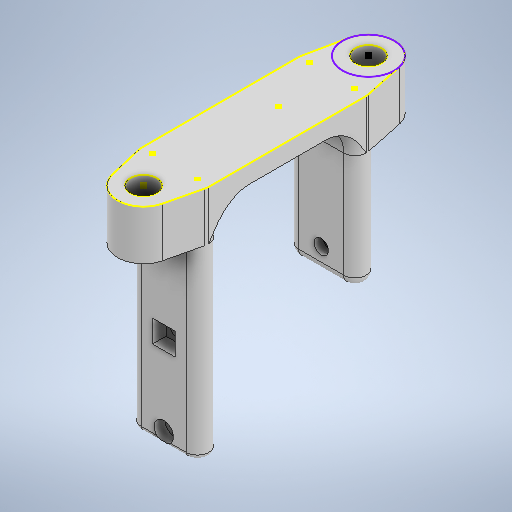
# Autodesk Inventor part: Latest_Odom
Saved by Autodesk Inventor 2025.1 (Build 291241020, 241B)
## iProperties
Created: 2024-11-18
Part Number: Latest_Odom
Material: Generic
Document SubType Name: Modeling
Designer: colli
Density: 1 g/cm^3
Appearance: Default
Author: colli
Autodesk Inventor part; units mm, degrees
ref_plane "YZ Plane" through (0, 0, 0) normal (1, 0, 0) x (0, 1, 0)
ref_plane "XZ Plane" through (0, 0, 0) normal (0, 1, 0) x (-1, 0, 0)
ref_plane "XY Plane" through (0, 0, 0) normal (0, 0, 1) x (1, 0, 0)
sketch "Sketch1" plane through (0, 0, 0) normal (0, 1, 0) x (-1, 0, 0)
  line L0 (1.833087, 41.275) -> (-1.833087, 41.275)
  line L1 (-1.833087, 41.275) -> (-3.666174, 38.1)
  line L2 (-3.666174, 38.1) -> (-1.833087, 34.925)
  line L3 (-1.833087, 34.925) -> (1.833087, 34.925)
  line L4 (1.833087, 34.925) -> (3.666174, 38.1)
  line L5 (3.666174, 38.1) -> (1.833087, 41.275)
  circle A0 centre (0, 38.1) radius 2.0955
  circle A1 centre (0, 38.1) radius 3.0353
  arc A2 (6.01682, 40.129871) -> (-6.01682, 40.129871) centre (0, 38.1) ccw
  line L6 (9.525, 29.21) -> (9.525, -15.24)
  line L7 (-9.525, 29.21) -> (-9.525, 19.812)
  circle A3 centre (0, 38.1) radius 3.81
  line L8 (-9.525, 19.812) -> (-9.525, 6.35)
  line L9 (9.525, 19.812) -> (9.525, 6.35)
  line L10 (0, 19.812) -> (0, -7.112) construction
  line L11 (0, 38.1) -> (0, 31.75)
  line L12 (9.525, -15.24) -> (9.525, 6.35)
  line L13 (-9.525, -15.24) -> (-9.525, 6.35)
  line L14 (1.833087, -28.575) -> (-1.833087, -28.575)
  line L15 (-1.833087, -28.575) -> (-3.666174, -25.4)
  line L16 (-3.666174, -25.4) -> (-1.833087, -22.225)
  line L17 (-1.833087, -22.225) -> (1.833087, -22.225)
  line L18 (1.833087, -22.225) -> (3.666174, -25.4)
  line L19 (3.666174, -25.4) -> (1.833087, -28.575)
  circle A4 centre (0, -25.4) radius 2.0955
  circle A5 centre (0, -25.4) radius 3.0353
  arc A6 (-6.01682, -27.429871) -> (6.01682, -27.429871) centre (0, -25.4) ccw
  line L20 (6.35, -12.065) -> (-6.35, -12.065)
  arc A7 (-6.35, -12.065) -> (-6.35, -18.415) centre (-6.35, -15.24) ccw
  arc A8 (6.35, -18.415) -> (6.35, -12.065) centre (6.35, -15.24) ccw
  line L21 (9.525, -15.24) -> (9.525, -7.112)
  line L22 (-9.525, -15.24) -> (-9.525, -7.112)
  circle A9 centre (0, -25.4) radius 3.81
  line L23 (0, -25.4) -> (0, -19.05)
  line L24 (6.35, -18.415) -> (-6.35, -18.415)
  line L25 (-6.01682, -27.429871) -> (-9.391765, -16.150106)
  line L26 (6.01682, -27.429871) -> (9.391765, -16.150106)
  line L27 (0, 31.115) -> (0, 32.385)
  line L28 (0, 32.385) -> (-6.35, 32.385)
  line L29 (0, 32.385) -> (6.35, 32.385)
  arc A10 (-6.35, 32.385) -> (-6.35, 26.035) centre (-6.35, 29.21) ccw
  line L30 (-6.35, 26.035) -> (6.35, 26.035)
  arc A11 (6.35, 26.035) -> (6.35, 32.385) centre (6.35, 29.21) ccw
  line L31 (-6.01682, 40.129871) -> (-9.35841, 30.224936)
  line L32 (6.01682, 40.129871) -> (9.35841, 30.224936)
  point P0 (0, 0)
  point P1 (-9.525, -16.51)
  point P2 (9.525, -16.51)
  dimension "d35" = 7.62
  dimension "d91" = 6.35
  dimension "d120" = 1.27
  constraints: 68 end point, 12 point on circle, 10 centre point, 5 tangent, 4 coincident, 2 horizontal, 2 point on line, 1 vertical, 12 other
  measures "d35" diameter of A3
  measures "d91" distance of L11.start L11.end
  measures "d120" distance of L27.start L27.end
extrude "Extrusion18" add sketch "Sketch1" along normal blind 5.08 contours A8 L24 A7 L20 | L26 A6 L25 A7 L24 A8
extrude "Extrusion19" add sketch "Sketch1" against normal blind 41.275 contours A8 L24 A7 L20
sketch "Sketch14" plane through (0, -41.275, 0) normal (0, -1, 0) x (1, 0, 0)
  arc A0 (-6.35, 31.115) -> (-6.35, 24.765) centre (-6.35, 27.94) ccw projected
  line L0 (-6.35, 24.765) -> (6.35, 24.765) projected
  arc A1 (6.35, 24.765) -> (6.35, 31.115) centre (6.35, 27.94) ccw projected
  line L1 (6.35, 31.115) -> (-6.35, 31.115) projected
  point P0 (0, 0)
extrude "Extrusion23" add sketch "Sketch14" along normal blind 20.472933
extrude "Extrusion26" add sketch "Sketch1" along normal up to surface (5.08 mm away) contours L32 A11 L29 L28 A10 L31 A2 | A11 L30 A10 L28 L29 | L6 A8 L20 A7 L13 L8 L7 A10 L30 A11
extrude "Extrusion27" add sketch "Sketch1" against normal up to surface (61.747933 mm away) contours A11 L30 A10 L28 L29
sketch "Sketch16" plane through (0, -61.747933, 0) normal (0, -1, 0) x (1, 0, 0)
  arc A0 (9.460852, 28.575) -> (6.35, 32.385) centre (6.35, 29.21) ccw
  line L0 (-6.35, 32.385) -> (6.35, 32.385)
  arc A1 (-6.35, 32.385) -> (-9.460852, 28.575) centre (-6.35, 29.21) ccw
  arc A2 (-9.460852, 28.575) -> (-6.35, 24.765) centre (-6.35, 27.94) ccw
  line L1 (-6.35, 24.765) -> (6.35, 24.765)
  arc A3 (6.35, 24.765) -> (9.460852, 28.575) centre (6.35, 27.94) ccw
  arc A4 (6.35, 26.035) -> (9.525, 29.21) centre (6.35, 29.21) ccw
  line L2 (6.35, 26.035) -> (-6.35, 26.035)
  arc A5 (-9.525, 29.21) -> (-6.35, 26.035) centre (-6.35, 29.21) ccw
  line L3 (-9.525, -15.24) -> (-9.525, 29.21)
  arc A6 (-6.35, -12.065) -> (-9.525, -15.24) centre (-6.35, -15.24) ccw
  line L4 (6.35, -12.065) -> (-6.35, -12.065)
  arc A7 (9.525, -15.24) -> (6.35, -12.065) centre (6.35, -15.24) ccw
  line L5 (9.525, 29.21) -> (9.525, -15.24)
  point P0 (0, 0)
extrude "Extrusion29" cut sketch "Sketch16" against normal blind 25.4 contours A3 L1 A2 A5 L2 A4
sketch "Sketch17" plane through (-6.35, -61.747933, 32.385) normal (0, 0, 1) x (1, 0, 0)
  line L0 (0, 0) -> (12.7, 0)
  line L1 (12.7, 61.747933) -> (12.7, 0)
  line L2 (0, 61.747933) -> (12.7, 61.747933)
  line L3 (0, 61.747933) -> (0, 0)
  line L4 (12.329967, 41.122933) -> (9.464987, 50.749947)
  arc A0 (9.464987, 50.749947) -> (3.235013, 50.749947) centre (6.35, 49.822933) ccw
  line L5 (3.235013, 50.749947) -> (0.370033, 41.122933)
  line L6 (0.370033, 12.522933) -> (3.235013, 2.89592)
  arc A1 (3.235013, 2.89592) -> (9.464987, 2.89592) centre (6.35, 3.822933) ccw
  line L7 (9.464987, 2.89592) -> (12.329967, 12.522933)
  circle A2 centre (6.35, 43.037933) radius 2.8
  circle A3 centre (6.35, 10.607933) radius 2.8
  circle A4 centre (6.35, 49.835433) radius 1.435
  circle A5 centre (6.35, 3.81) radius 1.435
  circle A6 centre (6.35, 26.822933) radius 2.032
  circle A7 centre (6.35, 49.835433) radius 2.7305
  line L8 (12.7, 20.472933) -> (15.875, 20.472933)
  line L9 (12.7, 20.472933) -> (0, 20.472933)
  line L10 (-3.175, 20.472933) -> (0, 20.472933)
  line L11 (-3.175, 20.472933) -> (-3.175, 66.827933)
  line L12 (0, 61.747933) -> (0, 20.472933)
  circle A8 centre (6.35, 26.822933) radius 2.032
  line L13 (0, 61.747933) -> (12.7, 61.747933)
  line L14 (0, 61.747933) -> (0, 20.472933)
  line L15 (12.7, 20.472933) -> (0, 20.472933)
  line L16 (12.7, 61.747933) -> (12.7, 20.472933)
  line L17 (15.875, 61.747933) -> (15.875, 66.827933)
  line L18 (15.741765, 66.827933) -> (15.875, 66.827933)
  line L19 (15.741765, 61.747933) -> (15.741765, 66.827933)
  line L20 (12.7, 61.747933) -> (15.741765, 61.747933)
  line L21 (12.7, 61.747933) -> (12.7, 20.472933)
  line L22 (12.7, 20.472933) -> (12.7, 20.472933)
  line L23 (12.7, 61.747933) -> (12.7, 20.472933)
  line L24 (6.35, 3.81) -> (6.35, 0)
  line L25 (6.35, 0) -> (-3.175, 0)
  line L26 (-3.175, 0) -> (-3.175, 20.472933)
  line L27 (6.35, 0) -> (15.875, 0)
  line L28 (15.875, 0) -> (15.875, 20.472933)
  circle A9 centre (6.35, 3.81) radius 2.7305
  line L29 (6.35, 26.822933) -> (6.35, 3.81)
  line L30 (6.35, 26.822933) -> (6.35, 49.835433)
  line L31 (15.875, 61.747933) -> (12.7, 61.747933)
  line L32 (6.35, 61.747933) -> (6.35, 26.822933)
  point P0 (6.35, 61.747933)
  dimension "d130" = 5.461
  dimension "d131" = 3.81
  dimension "d132" = 20.47293
  dimension "d133" = 5.461
  dimension "d134" = 34.925
  constraints: 58 end point, 10 centre point, 4 point on circle, 4 vertical, 3 perpendicular, 2 coincident, 1 horizontal
  measures "d130" diameter of A7
  measures "d131" distance of L24.start L24.end
  measures "d132" distance between parallel lines of L9 L27
  measures "d133" diameter of A9
  measures "d134" distance of L32.start L32.end
extrude "Extrusion30" cut sketch "Sketch17" along normal mid plane 25.4 contours L24 L29 A5 | A5 L29 L24
extrude "Extrusion31" cut sketch "Sketch17" along normal mid plane 25.4 contours L32 L30 A4 | A4 L30 L32
extrude "Extrusion32" cut sketch "Sketch17" against normal blind 3.048 contours L32 A4 L30 A7 | A7 L30 A4 L32 | L32 L30 A4 | A4 L30 L32
extrude "Extrusion33" cut sketch "Sketch17" against normal blind 3.048 contours A9 L29 A5 L24 | L24 A5 L29 A9 | L24 L29 A5 | A5 L29 L24
extrude "Extrusion34" cut sketch "Sketch17" along normal through all both and the other way through all contours L29 L30 A6 | A6 L30 L29
fillet "Fillet9" radius 8.89 6 edges at (-8.5951, 0, 26.9649) (8.5951, 0, 26.9649) (0, 0, 26.035) (-8.5951, 0, -12.9949) (8.5951, 0, -12.9949) (0, 0, -12.065)
sketch "Sketch18" plane through (-6.35, -61.747933, 32.385) normal (0, 0, 1) x (1, 0, 0)
  circle A0 centre (6.35, 26.822933) radius 2.032
  circle A1 centre (6.35, 3.81) radius 2.7305
  circle A2 centre (6.35, 49.835433) radius 2.7305
  line L0 (0, 0) -> (12.7, 0)
  line L1 (12.7, 61.747933) -> (12.7, 0)
  line L2 (0, 61.747933) -> (12.7, 61.747933)
  line L3 (0, 61.747933) -> (0, 0)
  line L4 (6.35, 26.822933) -> (6.35, 23.647933)
  line L5 (6.35, 23.647933) -> (9.525, 23.647933)
  line L6 (6.35, 26.822933) -> (6.35, 29.997933)
  line L7 (6.35, 29.997933) -> (3.175, 29.997933)
  line L8 (9.525, 23.647933) -> (3.175, 23.647933)
  line L9 (3.175, 23.647933) -> (3.175, 29.997933)
  line L10 (3.175, 29.997933) -> (9.525, 29.997933)
  line L11 (9.525, 29.997933) -> (9.525, 23.647933)
  point P0 (6.35, 61.747933)
  dimension "d146" = 3.175
  dimension "d147" = 3.175
  dimension "d148" = 3.175
  dimension "d149" = 3.175
  constraints: 16 end point, 3 perpendicular, 2 parallel, 2 vertical, 1 horizontal
  measures "d146" distance of L4.start L4.end
  measures "d147" distance of L4.end L5.end
  measures "d148" distance of L4.start L6.end
  measures "d149" distance of L6.end L7.end
extrude "Extrusion35" cut sketch "Sketch18" against normal blind 3.81 contours A0 L6 L10 L11 L5 L4 | A0 L4 L8 L9 L7 L6
sketch "Sketch19" plane through (6.35, 0, -18.415) normal (0, 0, -1) x (-1, 0, 0)
  circle A0 centre (6.35, -34.925) radius 2.032 projected
  line L0 (6.35, -34.925) -> (6.35, -38.1)
  line L1 (3.175, -38.1) -> (9.525, -38.1) projected
  line L2 (9.525, -38.1) -> (9.525, -31.75) projected
  line L3 (9.525, -31.75) -> (3.175, -31.75) projected
  line L4 (9.525, -38.1) -> (3.175, -38.1)
  line L5 (3.175, -38.1) -> (3.175, -31.75)
  line L6 (3.175, -31.75) -> (9.525, -31.75)
  line L7 (9.525, -31.75) -> (9.525, -38.1)
  point P0 (6.35, 0)
  constraints: 10 end point, 2 parallel, 1 horizontal, 1 midpoint, 1 perpendicular
extrude "Extrusion36" cut sketch "Sketch19" against normal blind 3.81
sketch "Sketch20" plane through (0, -61.747933, 0) normal (0, -1, 0) x (1, 0, 0)
  arc A0 (-6.35, 32.385) -> (-6.35, 26.035) centre (-6.35, 29.21) ccw projected
  line L0 (-6.35, 26.035) -> (6.35, 26.035) projected
  arc A1 (6.35, 26.035) -> (6.35, 32.385) centre (6.35, 29.21) ccw projected
  line L1 (-6.35, 32.385) -> (6.35, 32.385) projected
  point P0 (0, 0)
extrude "Extrusion37" add sketch "Sketch20" along normal blind 1.905
fillet "Fillet10" radius 2.54 8 edges at (-9.525, -63.6529, 29.21) (0, -63.6529, 26.035) (9.525, -63.6529, 29.21) (0, -63.6529, 32.385) (0, -41.275, -18.415) (9.525, -41.275, -15.24) (0, -41.275, -12.065) (-9.525, -41.275, -15.24)
sketch "Sketch21" plane through (0, 0, 0) normal (0, -1, 0) x (1, 0, 0)
  arc A0 (9.35841, 30.224936) -> (6.35, 32.385) centre (6.35, 29.21) ccw
  line L0 (6.01682, 40.129871) -> (9.35841, 30.224936)
  arc A1 (6.01682, 40.129871) -> (-6.01682, 40.129871) centre (0, 38.1) ccw
  line L1 (-9.35841, 30.224936) -> (-6.01682, 40.129871)
  arc A2 (-6.35, 32.385) -> (-9.35841, 30.224936) centre (-6.35, 29.21) ccw
  line L2 (-6.35, 32.385) -> (6.35, 32.385)
  circle A3 centre (0, 38.1) radius 3.81
  arc A4 (-9.391765, -16.150106) -> (-6.35, -18.415) centre (-6.35, -15.24) ccw
  line L3 (-6.01682, -27.429871) -> (-9.391765, -16.150106)
  arc A5 (-6.01682, -27.429871) -> (6.01682, -27.429871) centre (0, -25.4) ccw
  line L4 (9.391765, -16.150106) -> (6.01682, -27.429871)
  arc A6 (6.35, -18.415) -> (9.391765, -16.150106) centre (6.35, -15.24) ccw
  line L5 (6.35, -18.415) -> (-6.35, -18.415)
  circle A7 centre (0, -25.4) radius 3.81
  line L6 (0, 44.45) -> (0, 45.4025)
  arc A8 (7.107792, 39.77505) -> (-7.107792, 39.77505) centre (0, 38.1) ccw
  line L7 (9.35841, 30.224936) -> (6.01682, 40.129871)
  line L8 (9.35841, 30.224936) -> (7.107792, 39.77505)
  line L9 (-9.35841, 30.224936) -> (-7.107792, 39.77505)
  line L10 (0, -31.75) -> (0, -32.7025)
  arc A9 (-7.147551, -26.896334) -> (7.148285, -26.892828) centre (0, -25.4) ccw
  line L11 (9.391765, -16.150106) -> (7.148285, -26.892828)
  arc A10 (-9.525, -15.24) -> (-9.391765, -16.150106) centre (-6.35, -15.24) ccw
  line L12 (-9.491515, -15.699904) -> (-7.147551, -26.896334)
  point P0 (0, 0)
  point P1 (-9.412185, -16.078836)
  dimension "d157" = 0.9525
  dimension "d158" = 0.9525
  constraints: 12 end point, 9 point on circle, 4 tangent, 2 centre point, 2 coincident, 2 vertical
  measures "d157" distance of L6.start L6.end
  measures "d158" distance of L10.start L10.end
extrude "Extrusion38" add sketch "Sketch21" against normal up to surface (5.08 mm away) contours L0 A1 L6 A8 L8 | A1 L1 L9 A8 L6 | L3 A5 L10 A9 L12 A10 | A5 L4 L11 A9 L10
sketch "Sketch22" plane through (0, 0, 0) normal (0, -1, 0) x (1, 0, 0)
  arc A0 (9.35841, 30.224936) -> (6.35, 32.385) centre (6.35, 29.21) ccw
  line L0 (9.35841, 30.224936) -> (7.107792, 39.77505)
  arc A1 (7.107792, 39.77505) -> (-7.107792, 39.77505) centre (0, 38.1) ccw
  line L1 (-7.107792, 39.77505) -> (-9.35841, 30.224936)
  arc A2 (-6.35, 32.385) -> (-9.35841, 30.224936) centre (-6.35, 29.21) ccw
  line L2 (-6.35, 32.385) -> (6.35, 32.385)
  circle A3 centre (0, 38.1) radius 3.81
  arc A4 (-9.412185, -16.078836) -> (-6.35, -18.415) centre (-6.35, -15.24) ccw
  line L3 (-9.412185, -16.078836) -> (-7.147551, -26.896334)
  arc A5 (-7.147551, -26.896334) -> (7.148285, -26.892828) centre (0, -25.4) ccw
  line L4 (7.148285, -26.892828) -> (9.391765, -16.150106)
  arc A6 (6.35, -18.415) -> (9.391765, -16.150106) centre (6.35, -15.24) ccw
  line L5 (6.35, -18.415) -> (-6.35, -18.415)
  circle A7 centre (0, -25.4) radius 3.81
  circle A8 centre (0, -25.4) radius 3.7084
  circle A9 centre (0, 38.1) radius 3.7084
  point P0 (0, 0)
  dimension "d163" = 7.4168
  dimension "d164" = 7.4168
  constraints: 2 centre point, 2 coincident
  measures "d163" diameter of A8
  measures "d164" diameter of A9
extrude "Extrusion40" add sketch "Sketch22" against normal up to surface (5.08 mm away) contours A3 | A7
sketch "Sketch23" plane through (0, 0, 0) normal (0, -1, 0) x (1, 0, 0)
  arc A0 (-7.147551, -26.896334) -> (7.148285, -26.892828) centre (0, -25.4) ccw
  line L0 (-9.412185, -16.078836) -> (-7.147551, -26.896334)
  line L1 (7.148285, -26.892828) -> (9.391765, -16.150106)
  circle A1 centre (0, -25.4) radius 3.7084
  arc A2 (-9.412185, -16.078836) -> (-6.35, -18.415) centre (-6.35, -15.24) ccw
  line L2 (-9.412185, -16.078836) -> (-7.147551, -26.896334)
  arc A3 (-7.147551, -26.896334) -> (7.148285, -26.892828) centre (0, -25.4) ccw
  line L3 (7.148285, -26.892828) -> (9.391765, -16.150106)
  arc A4 (6.35, -18.415) -> (9.391765, -16.150106) centre (6.35, -15.24) ccw
  line L4 (6.35, -18.415) -> (-6.35, -18.415)
  circle A5 centre (0, 38.1) radius 3.7084
  arc A6 (9.35841, 30.224936) -> (6.35, 32.385) centre (6.35, 29.21) ccw
  line L5 (9.35841, 30.224936) -> (7.107792, 39.77505)
  arc A7 (7.107792, 39.77505) -> (-7.107792, 39.77505) centre (0, 38.1) ccw
  line L6 (-7.107792, 39.77505) -> (-9.35841, 30.224936)
  arc A8 (-6.35, 32.385) -> (-9.35841, 30.224936) centre (-6.35, 29.21) ccw
  line L7 (-6.35, 32.385) -> (6.35, 32.385)
  point P0 (0, 0)
extrude "Extrusion41" add sketch "Sketch23" along normal blind 8.89
sketch "Sketch24" plane through (-6.35, -61.112933, 32.385) normal (0, 0, 1) x (1, 0, 0)
  circle A0 centre (6.35, 49.200433) radius 2.7305
  circle A1 centre (6.35, 3.175) radius 2.7305
  line L0 (3.175, 29.362933) -> (9.525, 29.362933)
  line L1 (9.525, 29.362933) -> (9.525, 23.012933)
  line L2 (9.525, 23.012933) -> (3.175, 23.012933)
  line L3 (3.175, 23.012933) -> (3.175, 29.362933)
  line L4 (12.7, 52.222933) -> (0, 52.222933)
  line L5 (0, 52.222933) -> (0, 0)
  line L6 (12.7, 0) -> (0, 0)
  line L7 (12.7, 52.222933) -> (12.7, 0)
  line L8 (15.70841, 52.222933) -> (15.70841, 66.192933)
  line L9 (15.70841, 52.222933) -> (12.7, 52.222933)
  line L10 (12.7, 52.222933) -> (12.7, 0)
  line L11 (12.7, 0) -> (12.7, 0)
  line L12 (12.7, 52.222933) -> (12.7, 0)
  line L13 (15.875, 52.222933) -> (12.7, 52.222933)
  line L14 (15.875, 52.222933) -> (15.875, 66.192933)
  line L15 (15.875, 66.192933) -> (15.70841, 66.192933)
  line L16 (0, -2.54) -> (0, 0)
  line L17 (0, -2.54) -> (12.7, -2.54)
  line L18 (12.7, 0) -> (12.7, -2.54)
  line L19 (12.7, 0) -> (0, 0)
  line L20 (12.7, 0) -> (12.7, -2.54)
  line L21 (12.7, -2.54) -> (12.7, -2.54)
  line L22 (12.7, 0) -> (12.7, -2.54)
  line L23 (12.7, 0) -> (12.7, 0)
  line L24 (0, -2.54) -> (0, 0)
  line L25 (0, 0) -> (0, 0)
  line L26 (0, 0) -> (0, -2.54)
  line L27 (0, -2.54) -> (0, -2.54)
  line L28 (12.7, -2.54) -> (15.875, -2.54)
  line L29 (15.875, -2.54) -> (15.875, 0)
  line L30 (0, -2.54) -> (-3.175, -2.54)
  line L31 (-3.175, -2.54) -> (-3.175, 0)
  line L32 (-3.175, 0) -> (-3.175, 66.192933)
  line L33 (15.875, 0) -> (-3.175, 0)
  point P0 (6.35, 61.112933)
  point P1 (-3.175, 0)
  constraints: 10 end point, 3 horizontal, 1 perpendicular, 1 point on line
extrude "Extrusion42" cut sketch "Sketch24" along normal through all both and the other way through all contours L18 L17 L16 L6 | L33 L29 L28 L18 | L16 L30 L31 L33
fillet "Fillet11" radius 1.27 4 edges at (0, -61.1129, 26.035) (9.525, -61.1129, 29.21) (0, -61.1129, 32.385) (-9.525, -61.1129, 29.21)
sketch "Sketch25" plane through (0, 5.08, 0) normal (0, 1, 0) x (1, 0, 0)
  circle A0 centre (0, -38.1) radius 3.7084
  circle A1 centre (0, 25.4) radius 3.7084
  arc A2 (9.525, 15.24) -> (9.391765, 16.150106) centre (6.35, 15.24) ccw
  line L0 (7.148285, 26.892828) -> (9.391765, 16.150106)
  arc A3 (7.148285, 26.892828) -> (-7.147551, 26.896334) centre (0, 25.4) ccw
  line L1 (-9.412185, 16.078836) -> (-7.147551, 26.896334)
  arc A4 (-9.412185, 16.078836) -> (-9.525, 15.24) centre (-6.35, 15.24) ccw
  line L2 (-9.525, -29.21) -> (-9.525, 15.24)
  arc A5 (-9.525, -29.21) -> (-9.35841, -30.224936) centre (-6.35, -29.21) ccw
  line L3 (-7.107792, -39.77505) -> (-9.35841, -30.224936)
  arc A6 (-7.107792, -39.77505) -> (7.107792, -39.77505) centre (0, -38.1) ccw
  line L4 (9.35841, -30.224936) -> (7.107792, -39.77505)
  arc A7 (9.35841, -30.224936) -> (9.525, -29.21) centre (6.35, -29.21) ccw
  line L5 (9.525, 15.24) -> (9.525, -29.21)
  circle A8 centre (0, 25.4) radius 7.3025
  point P0 (0, 0)
  constraints: 1 centre point, 1 coincident
body "Solid2"
